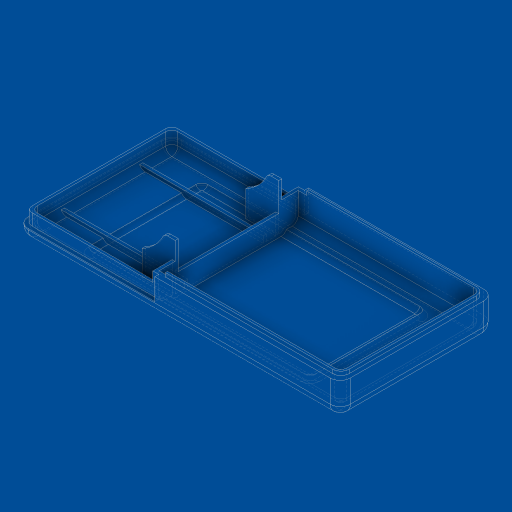
# Autodesk Inventor part: aus-200_bottom
Saved by Autodesk Inventor 2023.2 (Build 272271000, 271)
## iProperties
Created: 2023-01-27
Part Number: aus-200_bottom
Material: PC/ABS Plastic
Document SubType Name: Modeling
Designer: agmlego
Mass: 7.74771 g
Surface Area: 250.493 cm^2
Volume: 21.6857 cm^3
Density: 0.357273 g/cm^3
Appearance: Smooth - Black
Author: agmlego
Autodesk Inventor part; units mm, degrees
ref_plane "YZ Plane" through (0, 0, 0) normal (1, 0, 0) x (0, 1, 0)
ref_plane "XZ Plane" through (0, 0, 0) normal (0, 1, 0) x (-1, 0, 0)
ref_plane "XY Plane" through (0, 0, 0) normal (0, 0, 1) x (1, 0, 0)
sketch "Sketch1" plane through (0, 0, 0) normal (0, 1, 0) x (-1, 0, 0)
  line L0 (63.925, 30.5) -> (-63.925, 30.5)
  line L1 (-63.925, 30.5) -> (-63.925, -30.5)
  line L2 (-63.925, -30.5) -> (63.925, -30.5)
  line L3 (63.925, -30.5) -> (63.925, 30.5)
  line L4 (63.925, 0) -> (-63.925, 0) construction
  point P0 (0, 0)
  point P1 (0, 0)
  dimension "d0" = 61
  dimension "d1" = 127.85
  constraints: 10 end point, 3 midpoint, 2 parallel, 1 coincident, 1 horizontal, 1 perpendicular
  measures "d0" distance between parallel lines of L2 L0
  measures "d1" distance between parallel lines of L1 L3
extrude "Extrusion1" add sketch "Sketch1" along normal blind 13
fillet "Fillet1" radius 4 8 edges at (63.925, 6.5, 30.5) (0, 0, 30.5) (63.925, 0, 0) (63.925, 6.5, -30.5) (0, 0, -30.5) (-63.925, 6.5, -30.5) (-63.925, 0, 0) (-63.925, 6.5, 30.5)
sketch "Sketch2" plane through (0, 13, 0) normal (0, 1, 0) x (1, 0, 0)
  line L0 (61.305, -27.6) -> (-10.895, -27.6)
  line L1 (-10.895, -27.6) -> (-10.895, 27.6)
  line L2 (-10.895, 27.6) -> (61.305, 27.6)
  line L3 (61.305, 27.6) -> (61.305, -27.6)
  line L4 (61.305, 0) -> (63.925, 0) construction
  line L5 (63.925, -26.5) -> (63.925, 26.5) construction
  point P0 (0, 0)
  dimension "d5" = 55.2
  dimension "d6" = 2.62
  dimension "d7" = 72.2
  constraints: 10 end point, 2 midpoint, 2 parallel, 2 perpendicular, 1 horizontal
  measures "d5" distance of L2.end L0.start
  measures "d6" distance of L4.start L4.end
  measures "d7" distance of L0.start L0.end
extrude "Extrusion2" cut sketch "Sketch2" against normal blind 11.08
fillet "Fillet2" radius 2.4 5 edges at (25.205, 1.92, 27.6) (61.305, 7.46, 27.6) (61.305, 1.92, 0) (25.205, 1.92, -27.6) (61.305, 7.46, -27.6)
sketch "Sketch3" plane through (0, 13, 0) normal (0, 1, 0) x (1, 0, 0)
  line L0 (-10.895, 27.6) -> (58.905, 27.6) projected
  arc A0 (61.305, 25.2) -> (58.905, 27.6) centre (58.905, 25.2) ccw projected
  line L1 (61.305, 25.2) -> (61.305, -25.2) projected
  arc A1 (58.905, -27.6) -> (61.305, -25.2) centre (58.905, -25.2) ccw projected
  line L2 (58.905, -27.6) -> (-10.895, -27.6) projected
  line L3 (-10.895, 28.47) -> (58.905, 28.47)
  arc A2 (62.175, 25.2) -> (58.905, 28.47) centre (58.905, 25.2) ccw
  line L4 (62.175, 25.2) -> (62.175, -25.2)
  arc A3 (58.905, -28.47) -> (62.175, -25.2) centre (58.905, -25.2) ccw
  line L5 (58.905, -28.47) -> (-10.895, -28.47)
  line L6 (-7.475, 28.47) -> (-7.475, 27.6)
  line L7 (-7.475, -28.47) -> (-7.475, -27.6)
  line L8 (-10.895, -27.6) -> (58.905, -27.6) construction
  point P0 (0, 0)
  point P1 (-7.475, 28.035)
  dimension "d11" = 0.87
  dimension "d12" = 69.65
  constraints: 10 end point, 4 point on circle, 4 point on line, 2 centre point, 2 collinear, 1 midpoint, 1 perpendicular, 4 other
  measures "d11" distance between parallel lines of L0 L3
  measures "d12" distance from line of L4 point (-7.475, 28.035)
extrude "Extrusion3" add sketch "Sketch3" along normal blind 1.5
sketch "Sketch4" plane through (0, 13, 0) normal (0, 1, 0) x (1, 0, 0)
  line L0 (-12.095, 27.885) -> (-61.295, 27.885)
  line L1 (-61.295, 27.885) -> (-61.295, -27.885)
  line L2 (-61.295, -27.885) -> (-12.095, -27.885)
  line L3 (-12.095, -27.885) -> (-12.095, 27.885)
  line L4 (-10.895, -27.6) -> (-10.895, 27.6) construction
  line L5 (-10.895, 0) -> (-12.095, 0) construction
  point P0 (0, 0)
  dimension "d15" = 49.2
  dimension "d16" = 1.2
  dimension "d17" = 55.77
  constraints: 10 end point, 2 midpoint, 2 parallel, 2 perpendicular, 1 horizontal
  measures "d15" distance between parallel lines of L1 L3
  measures "d16" distance between parallel lines of L4 L3
  measures "d17" distance of L0.end L1.end
extrude "Extrusion4" cut sketch "Sketch4" against normal blind 11.29
fillet "Fillet3" radius 2.4 5 edges at (-36.695, 1.71, -27.885) (-61.295, 7.355, -27.885) (-61.295, 1.71, 0) (-36.695, 1.71, 27.885) (-61.295, 7.355, 27.885)
sketch "Sketch5" plane through (0, 13, 0) normal (0, 1, 0) x (1, 0, 0)
  line L0 (-59.925, -30.5) -> (59.925, -30.5) construction
  line L1 (-9.675, -30.5) -> (-9.675, -28.9)
  line L2 (-9.675, -30.5) -> (-59.925, -30.5)
  arc A0 (-63.925, -26.5) -> (-59.925, -30.5) centre (-59.925, -26.5) ccw construction
  arc A1 (-59.925, 30.5) -> (-63.925, 26.5) centre (-59.925, 26.5) ccw construction
  line L3 (-63.925, -26.5) -> (-63.925, 26.5)
  line L4 (-59.925, 30.5) -> (59.925, 30.5) construction
  line L5 (-59.925, 30.5) -> (-9.675, 30.5)
  line L6 (-9.675, 28.9) -> (-9.675, 30.5)
  line L7 (-9.675, 28.9) -> (-59.925, 28.9)
  line L8 (-59.925, 26.5) -> (-59.925, 30.5) construction
  line L9 (-63.925, 26.5) -> (-59.925, 26.5) construction
  line L10 (-62.325, 26.5) -> (-62.325, -26.5)
  line L11 (-9.675, -28.9) -> (-59.925, -28.9)
  arc A2 (-63.925, -26.5) -> (-59.925, -30.5) centre (-59.925, -26.5) ccw
  arc A3 (-62.325, -26.5) -> (-59.925, -28.9) centre (-59.925, -26.5) ccw
  line L12 (-63.925, 26.5) -> (-63.925, -26.5) construction
  arc A4 (-59.925, 30.5) -> (-63.925, 26.5) centre (-59.925, 26.5) ccw
  arc A5 (-59.925, 28.9) -> (-62.325, 26.5) centre (-59.925, 26.5) ccw
  point P0 (0, 0)
  dimension "d21" = 1.6
  dimension "d22" = 54.25
  constraints: 16 end point, 8 point on circle, 6 tangent, 4 centre point, 4 point on line, 3 collinear, 3 concentric, 3 vertical, 2 perpendicular, 1 horizontal
  measures "d21" distance of L1.start L1.end
  measures "d22" distance between parallel lines of L12 L1
extrude "Extrusion5" cut sketch "Sketch5" against normal blind 8.56
sketch "Sketch6" plane through (0, 13, 0) normal (0, 1, 0) x (1, 0, 0)
  line L0 (-9.675, 30.5) -> (-9.675, 28.9) construction
  line L1 (-9.675, 28.9) -> (-59.925, 28.9) projected
  arc A0 (-59.925, 28.9) -> (-62.325, 26.5) centre (-59.925, 26.5) ccw projected
  line L2 (-62.325, 26.5) -> (-62.325, -26.5) projected
  arc A1 (-62.325, -26.5) -> (-59.925, -28.9) centre (-59.925, -26.5) ccw projected
  line L3 (-59.925, -28.9) -> (-9.675, -28.9) projected
  line L4 (-9.675, -28.9) -> (-9.675, -30.5) construction
  line L5 (-9.675, -30.5) -> (59.925, -30.5) construction
  arc A2 (59.925, -30.5) -> (63.925, -26.5) centre (59.925, -26.5) ccw construction
  line L6 (63.925, -26.5) -> (63.925, 26.5) construction
  arc A3 (63.925, 26.5) -> (59.925, 30.5) centre (59.925, 26.5) ccw construction
  line L7 (59.925, 30.5) -> (-9.675, 30.5) construction
  line L8 (-7.475, -28.47) -> (-7.475, -27.6) construction
  line L9 (-7.475, -27.6) -> (-10.895, -27.6) projected
  line L10 (-10.895, -27.6) -> (-10.895, 27.6) projected
  line L11 (-10.895, 27.6) -> (-7.475, 27.6) projected
  line L12 (-7.475, 27.6) -> (-7.475, 28.47) construction
  line L13 (-7.475, 28.47) -> (58.905, 28.47) construction
  arc A4 (62.175, 25.2) -> (58.905, 28.47) centre (58.905, 25.2) ccw construction
  line L14 (62.175, 25.2) -> (62.175, -25.2) construction
  arc A5 (58.905, -28.47) -> (62.175, -25.2) centre (58.905, -25.2) ccw construction
  line L15 (58.905, -28.47) -> (-7.475, -28.47) construction
  line L16 (-12.095, -27.885) -> (-58.895, -27.885) projected
  arc A6 (-61.295, -25.485) -> (-58.895, -27.885) centre (-58.895, -25.485) ccw projected
  line L17 (-61.295, -25.485) -> (-61.295, 25.485) projected
  arc A7 (-58.895, 27.885) -> (-61.295, 25.485) centre (-58.895, 25.485) ccw projected
  line L18 (-58.895, 27.885) -> (-12.095, 27.885) projected
  line L19 (-12.095, 27.885) -> (-12.095, -27.885) projected
  line L20 (-12.095, -27.885) -> (-58.895, -27.885) construction
  line L21 (-12.095, -27.885) -> (-12.095, -28.9)
  line L22 (-59.925, -28.9) -> (-9.675, -28.9) construction
  line L23 (-12.095, 27.885) -> (-12.095, 28.9)
  line L24 (-9.675, 28.9) -> (-59.925, 28.9) construction
  point P0 (0, 0)
  constraints: 4 end point, 2 point on line, 1 perpendicular, 1 vertical
extrude "Extrusion6" cut sketch "Sketch6" against normal blind 3.96 contours L23 L18 A7 L17 A6 L16 L21 L3 A1 L2 A0 L1
sketch "Sketch7" plane through (0, 0, 0) normal (0, -1, 0) x (1, 0, 0)
  line L0 (-46, -24.5) -> (46, -24.5)
  line L1 (46, -24.5) -> (46, 24.5)
  line L2 (46, 24.5) -> (-46, 24.5)
  line L3 (-46, 24.5) -> (-46, -24.5)
  line L4 (0, -24.5) -> (0, 24.5) construction
  point P0 (0, 0)
  point P1 (0, 0)
  dimension "d27" = 49
  dimension "d28" = 92
  constraints: 10 end point, 3 midpoint, 2 parallel, 1 coincident, 1 horizontal, 1 perpendicular
  measures "d27" distance of L2.end L0.start
  measures "d28" distance of L0.start L0.end
extrude "Extrusion7" add sketch "Sketch7" along normal blind 0.8
fillet "Fillet4" radius 4 4 edges at (-46, -0.4, -24.5) (46, -0.4, -24.5) (-46, -0.4, 24.5) (46, -0.4, 24.5)
fillet "Fillet5" radius 4 8 edges at (44.8284, -0.8, 23.3284) (0, -0.8, 24.5) (-44.8284, -0.8, 23.3284) (-46, -0.8, 0) (-44.8284, -0.8, -23.3284) (0, -0.8, -24.5) (44.8284, -0.8, -23.3284) (46, -0.8, 0)
sketch "Sketch8" plane through (0, 1.92, 0) normal (0, 1, 0) x (1, 0, 0)
  line L0 (-44.5, 23) -> (44.5, 23)
  line L1 (44.5, 23) -> (44.5, -23)
  line L2 (44.5, -23) -> (-44.5, -23)
  line L3 (-44.5, -23) -> (-44.5, 23)
  line L4 (0, 23) -> (0, -23) construction
  point P0 (0, 0)
  point P1 (0, 0)
  dimension "d33" = 46
  dimension "d34" = 89
  constraints: 10 end point, 3 midpoint, 2 parallel, 1 coincident, 1 horizontal, 1 perpendicular
  measures "d33" distance of L2.end L0.start
  measures "d34" distance of L0.start L0.end
extrude "Extrusion8" cut sketch "Sketch8" against normal blind 1.36
fillet "Fillet6" radius 2.4 4 edges at (-44.5, 1.135, -23) (-44.5, 1.135, 23) (44.5, 1.24, 23) (44.5, 1.24, -23)
sketch "Sketch9" plane through (0, 1.92, 0) normal (0, -1, 0) x (1, 0, 0)
  line L0 (-10.895, 23) -> (-10.895, -23) projected
  line L1 (-12.095, 23) -> (-10.895, 23) projected
  line L2 (-12.095, -23) -> (-12.095, 23) projected
  line L3 (-10.895, -23) -> (-12.095, -23) projected
  point P0 (0, 0)
extrude "Extrusion9" add sketch "Sketch9" along normal up to surface (1.36 mm away)
fillet "Fillet7" radius 2.4 10 edges at (-43.7971, 0.56, 22.2971) (-44.5, 0.56, 0) (-43.7971, 0.56, -22.2971) (-27.0975, 0.56, -23) (-27.0975, 0.56, 23) (43.7971, 0.56, 22.2971) (44.5, 0.56, 0) (43.7971, 0.56, -22.2971) (15.6025, 0.56, -23) (15.6025, 0.56, 23)
sketch "Sketch10" plane through (0, 0.56, 0) normal (0, 1, 0) x (1, 0, 0)
  line L0 (-10.895, -27.6) -> (-10.895, 27.6) construction
  line L1 (-10.895, -21.185) -> (-24.045, -21.185)
  line L2 (-24.045, -21.185) -> (-24.045, -19.935)
  line L3 (-24.045, -19.935) -> (-10.895, -19.935)
  line L4 (-10.895, -19.935) -> (-10.895, -21.185)
  line L5 (-10.895, 21.185) -> (-24.045, 21.185)
  line L6 (-24.045, 21.185) -> (-24.045, 19.935)
  line L7 (-24.045, 19.935) -> (-10.895, 19.935)
  line L8 (-10.895, 19.935) -> (-10.895, 21.185)
  line L9 (-10.895, -19.935) -> (-10.895, 19.935) construction
  point P0 (0, 0)
  point P1 (-10.895, 0)
  dimension "d41" = 1.25
  dimension "d42" = 39.87
  dimension "d43" = 13.15
  constraints: 18 end point, 4 parallel, 2 collinear, 2 horizontal, 2 midpoint, 2 perpendicular, 2 point on line, 1 vertical
  measures "d41" distance of L1.end L2.end
  measures "d42" distance between parallel lines of L7 L3
  measures "d43" distance of L2.end L3.end
extrude "Extrusion10" add sketch "Sketch10" along normal blind 19.65
sketch "Sketch11" plane through (-10.895, 20.21, -21.185) normal (0, 0, -1) x (-1, 0, 0)
  line L0 (0, 0) -> (13.15, 0) construction
  arc A0 (4.32, 0) -> (13.15, -9.3186) centre (22.128, 8.0315) ccw
  line L1 (13.15, -19.6386) -> (13.15, 0) construction
  line L2 (4.32, 0) -> (13.15, 0)
  line L3 (13.15, 0) -> (13.15, -9.3186)
  line L4 (0, -7.21) -> (0, 0) construction
  line L5 (1.2, -7.21) -> (0, -7.21) construction
  line L6 (0, -7.21) -> (7.9477, -5.4053) construction
  point P0 (-10.895, -20.21)
  dimension "d46" = 4.32
  dimension "d47" = 10.32
  dimension "d48" = 8.15
  constraints: 6 end point, 3 point on circle, 1 centre point, 1 collinear, 1 perpendicular, 1 point on line
  measures "d46" distance from line of L4 L2.start
  measures "d47" distance of L1.start L3.end
  measures "d48" distance of L4.start L6.end
extrude "Extrusion11" cut sketch "Sketch11" against normal through all
fillet "Fillet8" radius 2 2 edges at (-15.215, 20.21, 20.56) (-15.215, 20.21, -20.56)
sketch "Sketch12" plane through (-12.095, 13, -19.935) normal (-1, 0, 0) x (0, 0, 1)
  line L0 (39.87, -12.44) -> (39.87, 0) construction
  line L1 (0, 0) -> (39.87, 0)
  line L2 (39.87, 0) -> (39.87, -4.14)
  line L3 (39.87, -4.14) -> (0, -4.14)
  line L4 (0, -4.14) -> (0, 0)
  line L5 (39.87, -12.44) -> (0, -12.44) construction
  point P0 (19.935, -13)
  dimension "d52" = 8.3
  constraints: 8 end point, 2 parallel, 1 horizontal, 1 perpendicular, 1 point on line
  measures "d52" distance between parallel lines of L5 L3
extrude "Extrusion12" cut sketch "Sketch12" against normal up to surface (1.2 mm away)
sketch "Sketch13" plane through (0, 0.56, 0) normal (0, 1, 0) x (1, 0, 0)
  line L0 (-12.095, -19.935) -> (-12.095, 19.935) construction
  line L1 (-61.295, 25.485) -> (-61.295, -25.485) construction
  line L2 (-12.095, -16.175) -> (-61.295, -16.175)
  line L3 (-61.295, -16.175) -> (-61.295, -14.915)
  line L4 (-61.295, -14.915) -> (-12.095, -14.915)
  line L5 (-12.095, -14.915) -> (-12.095, -16.175)
  line L6 (-12.095, 16.175) -> (-61.295, 16.175)
  line L7 (-61.295, 16.175) -> (-61.295, 14.915)
  line L8 (-61.295, 14.915) -> (-12.095, 14.915)
  line L9 (-12.095, 14.915) -> (-12.095, 16.175)
  line L10 (-12.095, -14.915) -> (-12.095, 14.915) construction
  line L11 (-12.095, -19.935) -> (-12.095, 19.935) construction
  point P0 (0, 0)
  point P1 (-12.095, 0)
  dimension "d55" = 1.26
  dimension "d56" = 29.83
  constraints: 18 end point, 4 parallel, 4 point on line, 3 perpendicular, 2 horizontal, 2 midpoint, 1 collinear
  measures "d55" distance between parallel lines of L8 L6
  measures "d56" distance between parallel lines of L4 L8
extrude "Extrusion13" add sketch "Sketch13" along normal blind 2.58
body "Solid1"
